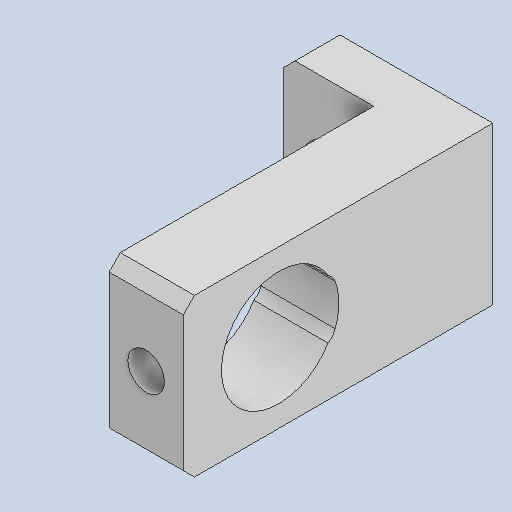
# Autodesk Inventor part: shutter-mount
Saved by Autodesk Inventor 2024.2 (Build 282272000, 272)
## iProperties
Created: 2021-03-22
Part Number: shutter-mount
Material: Generic
Document SubType Name: Modeling
Designer: maria
Density: 1 g/cm^3
Appearance: Default
Author: maria
Autodesk Inventor part; units mm, degrees
note: some values were not read from the file. Chosen so that the rebuilt part matches the saved one: direction of "Hole3".
ref_plane "YZ Plane" through (0, 0, 0) normal (1, 0, 0) x (0, 1, 0)
ref_plane "XZ Plane" through (0, 0, 0) normal (0, 1, 0) x (-1, 0, 0)
ref_plane "XY Plane" through (0, 0, 0) normal (0, 0, 1) x (1, 0, 0)
sketch "Sketch1" plane through (0, 0, 0) normal (0, 0, 1) x (1, 0, 0)
  line L0 (-4, 7) -> (4, 7)
  line L1 (4, 7) -> (4, -7)
  line L2 (4, -7) -> (-4, -7)
  line L3 (-4, -7) -> (-4, 7)
  point P0 (0, 0)
  dimension "WIDTH" = 14
  dimension "d1" = 7
  dimension "d2" = 4
  dimension "LENGTH" = 8
  constraints: 8 end point, 2 parallel, 1 horizontal, 1 perpendicular
  measures "WIDTH" distance of L2.end L0.start
  measures "d1" distance from line of point (0, 0) L0
  measures "d2" distance from line of point (0, 0) L1
  measures "LENGTH" distance of L0.start L0.end
extrude "Extrusion1" add sketch "Sketch1" along normal blind 4
sketch "Sketch2" plane through (0, 0, 4) normal (0, 0, 1) x (1, 0, 0)
  line L0 (0, -3.0354) -> (0, -0.0354) construction
  line L1 (2.25, -3.0354) -> (2.25, -0.0354)
  line L2 (-2.25, -0.0354) -> (-2.25, -3.0354)
  arc A0 (-2.25, -3.0354) -> (2.25, -3.0354) centre (0, -3.0354) ccw
  arc A1 (2.25, -0.0354) -> (-2.25, -0.0354) centre (0, -0.0354) ccw
  point P0 (0, -1.5354)
  point P1 (0, 0)
  dimension "d44" = 0
  dimension "d45" = 1.5354
  dimension "d55" = 2.25
  dimension "d56" = 3
  constraints: 8 end point, 4 point on circle, 4 tangent, 2 centre point, 1 midpoint, 1 parallel, 1 vertical
  measures "d44" horizontal distance of point (0, 0) point (0, -1.535)
  measures "d45" distance of point (0, -1.535) point (0, 0)
  measures "d55" radius of A1
  measures "d56" distance of L0.start L0.end
extrude "Extrusion3" cut sketch "Sketch2" against normal through all
sketch "Sketch3" plane through (0, 0, 0) normal (0, 0, 1) x (1, 0, 0)
  line L0 (4, 7) -> (10.6, 7)
  line L1 (10.6, 7) -> (10.6, -7)
  line L2 (10.6, -7) -> (4, -7)
  line L3 (4, -7) -> (4, 7)
  line L4 (4, -7) -> (4, 7) projected
  line L5 (4, 7) -> (-4, 7) projected
  point P0 (0, 0)
  dimension "d15" = 0
  dimension "d16" = 0
  dimension "d17" = 6.6
  dimension "d18" = 14
  constraints: 8 end point, 2 parallel, 1 horizontal, 1 perpendicular
  measures "d15" distance between parallel lines of L4 L3
  measures "d16" distance between parallel lines of L5 L0
  measures "d17" distance of L0.start L0.end
  measures "d18" distance of L0.end L1.end
extrude "Extrusion2" add sketch "Sketch3" along normal blind 27.55
sketch "Sketch4" plane through (10.6, -7, 0) normal (1, 0, 0) x (0, 0, -1)
  point P0 (0, 7)
  point P1 (-19.05, 7)
  dimension "d28" = 0
  dimension "d29" = 19.05
  measures "d28" vertical distance of point (0, 7) point (-19.05, 7)
  measures "d29" distance of point (0, 7) point (-19.05, 7)
hole "Hole2" at (10.6, 0, 19.05) direction (-1, 0, 0) diameter 10.2 end through all
sketch "Sketch5" plane through (0, 0, 27.55) normal (0, 0, 1) x (1, 0, 0)
  line L0 (10.6, -7) -> (10.6, 7) projected
  point P0 (0, 0)
  point P1 (7.3, 0)
  dimension "d37" = 0
  dimension "d38" = 3.3
  measures "d37" vertical distance of point (0, 0) point (7.3, 0)
  measures "d38" distance from line of point (7.3, 0) L0
hole "Hole3" at (7.3, 0, 27.55) direction (0, 0, -1) diameter 3.2639 end up to surface
chamfer "Chamfer1" distance 1 angle 45 4 edges at (7.3, 7, 27.55) (7.3, -7, 27.55) (-4, -7, 2) (-4, 7, 2)
sketch "Sketch7" plane through (10.6, -7, 0) normal (1, 0, 0) x (0, 0, -1)
  circle A0 centre (-19.05, 7) radius 5.35
  circle A1 centre (-19.05, 7) radius 5.1 projected
  circle A2 centre (-15.4322, 5.6832) radius 1.5
  circle A3 centre (-15.4322, 8.3168) radius 1.5
  line L0 (-15.4322, 5.6832) -> (-19.05, 7)
  line L1 (-19.05, 7) -> (-15.4322, 8.3168)
  line L2 (-19.05, 7) -> (-13.7, 7)
  point P0 (0, 7)
  point P1 (-14.0226, 8.8298)
  point P2 (-14.6664, 9.6066)
  point P3 (-14.6664, 4.3934)
  point P4 (-14.0226, 5.1702)
  dimension "d61" = 10.7
  dimension "d59" = 0
  dimension "d60" = 0
  dimension "d62" = 3
  dimension "d63" = 3
  dimension "d65" = 3.85
  dimension "d66" = 3.85
  dimension "d67" = 20
  dimension "d68" = 20
  constraints: 6 end point, 2 centre point, 1 horizontal, 3 other
  measures "d59" distance of L0.end point (-19.05, 7)
  measures "d60" distance of L0.end point (-19.05, 7)
  measures "d62" diameter of A2
  measures "d63" diameter of A3
  measures "d65" distance of point (-19.05, 7) L0.start
  measures "d66" distance of point (-19.05, 7) L1.end
  measures "d67" angle of L1 L2
  measures "d68" angle of L2 L0
extrude "Extrusion4" cut sketch "Sketch7" against normal through all contours L2 A1 A3 A0 | A0 A2 A1 L2 | A3 A1 | A2 A1
equation "\"d1\" = 0.5 * WIDTH"
equation "\"d2\" = 0.5 * LENGTH"
equation "\"d18\" = WIDTH"
equation "\"d29\" = BEAM_HEIGHT"
equation "\"d38\" = 0.5 * d17"
equation "\"d65\" = 0.5 * d61 - 0.5 * d62"
equation "\"d66\" = 0.5 * d61 - 0.5 * d62"
equation "\"BEAM_HEIGHT\" = 19.05"
body "Solid1"
